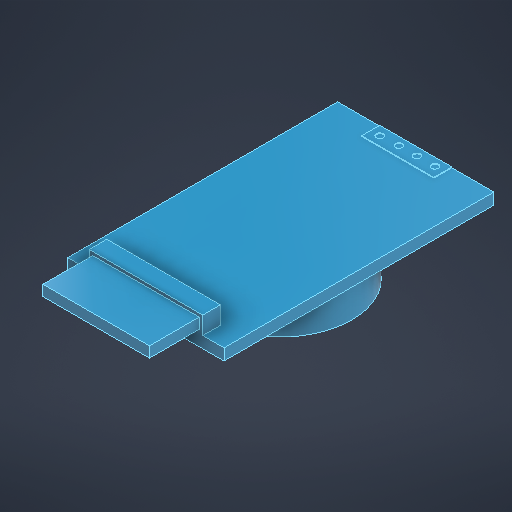
# Autodesk Inventor part: ZS042
Saved by Autodesk Inventor 2025.2 (Build 292293000, 293)
## iProperties
Created: 2026-01-02
Part Number: ZS042
Material: PC/ABS Plastic
Document SubType Name: Modeling
Designer: sam
Density: 1.1 g/cm^3
Appearance: Sky Blue Dark
Author: sam
Autodesk Inventor part; units mm, degrees
ref_plane "YZ Plane" through (0, 0, 0) normal (1, 0, 0) x (0, 1, 0)
ref_plane "XZ Plane" through (0, 0, 0) normal (0, 1, 0) x (-1, 0, 0)
ref_plane "XY Plane" through (0, 0, 0) normal (0, 0, 1) x (1, 0, 0)
sketch "Sketch1" plane through (0, 0, 0) normal (0, 1, 0) x (-1, 0, 0)
  line L0 (11, -19) -> (-11, -19)
  line L1 (-11, -19) -> (-11, 19)
  line L2 (-11, 19) -> (11, 19)
  line L3 (11, 19) -> (11, -19)
  line L4 (11, -19) -> (-11, 19) construction
  line L5 (-11, -19) -> (11, 19) construction
  point P0 (0, 0)
  dimension "d0" = 22
  dimension "d1" = 38
  constraints: 12 end point, 2 midpoint, 2 parallel, 1 horizontal, 1 perpendicular
  measures "d0" distance of L1.end L2.end
  measures "d1" distance of L0.end L1.end
extrude "Extrusion1" add sketch "Sketch1" along normal blind 1.6
sketch "Sketch2" plane through (0, 0, 0) normal (0, -1, 0) x (1, 0, 0)
  circle A0 centre (0, 0) radius 10
  circle A1 centre (0, 0) radius 9
  line L0 (-4, 9) -> (-4, 9)
  line L1 (-4, 9) -> (-4, 11)
  line L2 (-4, 11) -> (4, 11)
  line L3 (4, 11) -> (4, 9)
  point P0 (-4, 9.1652)
  point P1 (4, 9.1652)
  dimension "d4" = 20
  dimension "d7" = 18
  dimension "d8" = 8
  dimension "d9" = 2
  dimension "d10" = 0
  constraints: 8 end point, 2 centre point, 2 coincident, 2 parallel, 1 horizontal, 1 midpoint, 1 perpendicular
  measures "d4" diameter of A0
  measures "d7" diameter of A1
  measures "d8" distance of L1.end L2.end
  measures "d9" distance of L0.end L1.end
  measures "d10" distance of L0.start point (-4, 9)
extrude "Extrusion2" add sketch "Sketch2" along normal blind 5
sketch "Sketch3" plane through (0, 1.6, 0) normal (0, 1, 0) x (1, 0, 0)
  line L0 (-11, -19) -> (11, -19) projected
  line L1 (-8, -19) -> (8, -19)
  line L2 (8, -19) -> (8, -16.5)
  line L3 (8, -16.5) -> (-8, -16.5)
  line L4 (-8, -16.5) -> (-8, -19)
  line L5 (-11, 19) -> (-11, -19) projected
  line L6 (11, -19) -> (11, 19) projected
  point P0 (0, 0)
  dimension "d11" = 2.5
  dimension "d12" = 3
  dimension "d13" = 3
  constraints: 8 end point, 2 parallel, 1 horizontal, 1 perpendicular, 1 point on line
  measures "d11" distance of L2.end L1.end
  measures "d12" distance between parallel lines of L5 L4
  measures "d13" distance between parallel lines of L6 L2
extrude "Extrusion3" add sketch "Sketch3" along normal blind 2.5
sketch "Sketch4" plane through (0, 1.6, 0) normal (0, 1, 0) x (1, 0, 0)
  line L0 (11, 19) -> (-11, 19) projected
  line L1 (-5.0746, 19) -> (5.08, 19)
  line L2 (5.08, 19) -> (5.08, 16.46)
  line L3 (5.08, 16.46) -> (-5.0746, 16.46)
  line L4 (-5.0746, 16.46) -> (-5.0746, 19)
  line L5 (-11, 19) -> (-11, -19) projected
  line L6 (11, -19) -> (11, 19) projected
  circle A0 centre (-3.8046, 17.73) radius 0.5
  circle A1 centre (-1.27, 17.8958) radius 0.5
  circle A2 centre (1.27, 17.8958) radius 0.5
  circle A3 centre (3.81, 17.8958) radius 0.5
  point P0 (0, 0)
  point P1 (0.0027, 19)
  point P2 (0, 19)
  dimension "d16" = 2.54
  dimension "d19" = 1
  dimension "d20" = 1
  dimension "d21" = 1
  dimension "d22" = 1
  dimension "d23" = 2.54
  dimension "d24" = 2.54
  dimension "d25" = 2.54
  dimension "d26" = 1.27
  dimension "d27" = 1.27
  dimension "d29" = 1.27
  dimension "d30" = 1.27
  constraints: 8 end point, 4 centre point, 2 midpoint, 2 parallel, 1 horizontal, 1 perpendicular, 1 point on line
  measures "d16" distance of L1.end L2.end
  measures "d19" diameter of A0
  measures "d20" diameter of A1
  measures "d21" diameter of A2
  measures "d22" diameter of A3
  measures "d23" distance of A1.centre A2.centre
  measures "d24" distance of A3.centre A2.centre
  measures "d25" distance of A0.centre A1.centre
  measures "d26" distance from line of L4 A0.centre
  measures "d27" distance from line of L2 A3.centre
  measures "d29" horizontal distance of point (0, 19) A2.centre
  measures "d30" distance from line of L3 A0.centre
extrude "Extrusion4" add sketch "Sketch4" along normal blind 0.1
sketch "Sketch5" plane through (-11, 0, 19) normal (0, 0, 1) x (1, 0, 0)
  line L0 (3.5, 3.6) -> (18.5, 3.6)
  line L1 (18.5, 3.6) -> (18.5, 2.1)
  line L2 (18.5, 2.1) -> (3.5, 2.1)
  line L3 (3.5, 2.1) -> (3.5, 3.6)
  line L4 (3, 4.1) -> (19, 4.1) projected
  line L5 (3, 1.6) -> (3, 4.1) projected
  line L6 (19, 1.6) -> (19, 4.1) projected
  line L7 (0, 1.6) -> (3, 1.6) projected
  point P0 (11, 0)
  dimension "d35" = 0.5
  dimension "d36" = 0.5
  dimension "d37" = 0.5
  dimension "d38" = 0.5
  constraints: 8 end point, 2 parallel, 1 horizontal, 1 perpendicular
  measures "d35" distance between parallel lines of L4 L0
  measures "d36" distance between parallel lines of L5 L3
  measures "d37" distance between parallel lines of L6 L1
  measures "d38" distance between parallel lines of L7 L2
extrude "Extrusion5" add sketch "Sketch5" along normal blind 7
equation "\"d13\" = d12"
body "Solid1"
